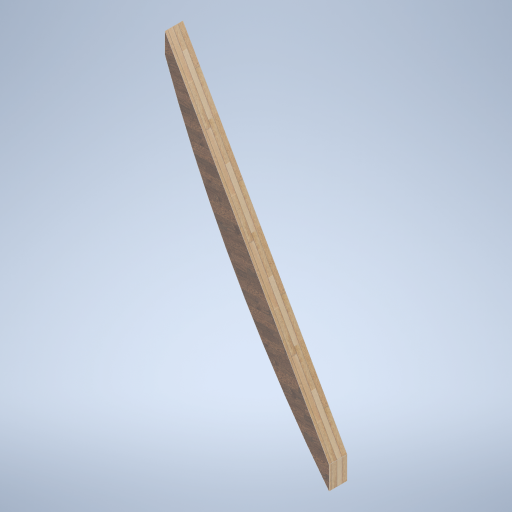
# Autodesk Inventor part: side_curve_beam_04
Saved by Autodesk Inventor 2024.2 (Build 282272000, 272)
## iProperties
Created: 2024-05-24
Part Number: side_curve_beam_04
Material: Wood (Maple)
Document SubType Name: Modeling
Designer: LOSTER_1
Density: 0.67 g/cm^3
Appearance: Natural Maple - Glossy Dark Tint
Author: LOSTER_1
Autodesk Inventor part; units mm, degrees
ref_plane "YZ Plane" through (0, 0, 0) normal (1, 0, 0) x (0, 1, 0)
ref_plane "XZ Plane" through (0, 0, 0) normal (0, 1, 0) x (-1, 0, 0)
ref_plane "XY Plane" through (0, 0, 0) normal (0, 0, 1) x (1, 0, 0)
sketch "Sketch1" plane through (0, 0, 0) normal (0, 0, 1) x (1, 0, 0)
  line L0 (944.5906, -1536.2377) -> (-871.9078, 1711.4549)
  line L1 (944.5906, -1668.3747) -> (944.5906, -1536.2377)
  line L2 (944.5906, -1536.2377) -> (944.5906, -1791.3892)
  line L3 (-871.9078, 1484.5818) -> (-871.9078, 1711.4549)
  arc A0 (-871.9078, 1484.5818) -> (944.5906, -1791.3892) centre (10402.3503, 5594.4609) ccw
  point P0 (0, 0)
  point P1 (963.6736, -1791.3892)
  point P2 (-975.9036, 1415.1228)
  point P3 (-975.579, 1678.3612)
  dimension "d3" = 12000
  constraints: 8 end point, 2 point on circle, 1 centre point, 1 point on line, 1 vertical
  measures "d3" radius of A0
extrude "Extrusion2" add sketch "Sketch1" along normal blind 200
body "Solid2"
